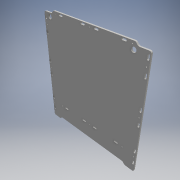
# Autodesk Inventor part: painel direito
Saved by Autodesk Inventor 2016 (Build 200138000, 138)
## iProperties
Created: 2016-08-08
Part Number: painel direito
Material: Generic
Document SubType Name: Modeling
Designer: Waldo
Density: 1 g/cm^3
Appearance: Default
Author: Waldo
Autodesk Inventor part; units mm, degrees
ref_plane "YZ Plane" through (0, 0, 0) normal (1, 0, 0) x (0, 1, 0)
ref_plane "XZ Plane" through (0, 0, 0) normal (0, 1, 0) x (-1, 0, 0)
ref_plane "XY Plane" through (0, 0, 0) normal (0, 0, 1) x (1, 0, 0)
sketch "Sketch1" plane through (0, 0, 0) normal (0, 1, 0) x (-1, 0, 0)
  line L0 (173.9968, 182.2069) -> (173.9968, 192.2069)
  arc A0 (167.7968, 182.2069) -> (173.9968, 182.2069) centre (170.8968, 182.2069) ccw
  line L1 (167.7968, 192.2069) -> (167.7968, 182.2069)
  arc A1 (173.9968, 192.2069) -> (167.7968, 192.2069) centre (170.8968, 192.2069) ccw
  line L2 (14.5968, -131.4908) -> (4.5968, -131.4908)
  arc A2 (14.5968, -137.6908) -> (14.5968, -131.4908) centre (14.5968, -134.5908) ccw
  line L3 (4.5968, -137.6908) -> (14.5968, -137.6908)
  arc A3 (4.5968, -131.4908) -> (4.5968, -137.6908) centre (4.5968, -134.5908) ccw
  line L4 (105.0968, -131.4908) -> (95.0968, -131.4908)
  arc A4 (105.0968, -137.6908) -> (105.0968, -131.4908) centre (105.0968, -134.5908) ccw
  line L5 (95.0968, -137.6908) -> (105.0968, -137.6908)
  arc A5 (95.0968, -131.4908) -> (95.0968, -137.6908) centre (95.0968, -134.5908) ccw
  line L6 (-135.9032, -137.6908) -> (-125.9032, -137.6908)
  arc A6 (-135.9032, -131.4908) -> (-135.9032, -137.6908) centre (-135.9032, -134.5908) ccw
  line L7 (-125.9032, -131.4908) -> (-135.9032, -131.4908)
  arc A7 (-125.9032, -137.6908) -> (-125.9032, -131.4908) centre (-125.9032, -134.5908) ccw
  line L8 (-45.4032, -137.6908) -> (-35.4032, -137.6908)
  arc A8 (-45.4032, -131.4908) -> (-45.4032, -137.6908) centre (-45.4032, -134.5908) ccw
  line L9 (-35.4032, -131.4908) -> (-45.4032, -131.4908)
  arc A9 (-35.4032, -137.6908) -> (-35.4032, -131.4908) centre (-35.4032, -134.5908) ccw
  line L10 (14.5968, 210.5092) -> (4.5968, 210.5092)
  arc A10 (14.5968, 204.3092) -> (14.5968, 210.5092) centre (14.5968, 207.4092) ccw
  line L11 (4.5968, 204.3092) -> (14.5968, 204.3092)
  arc A11 (4.5968, 210.5092) -> (4.5968, 204.3092) centre (4.5968, 207.4092) ccw
  line L12 (105.0968, 210.5092) -> (95.0968, 210.5092)
  arc A12 (105.0968, 204.3092) -> (105.0968, 210.5092) centre (105.0968, 207.4092) ccw
  line L13 (95.0968, 204.3092) -> (105.0968, 204.3092)
  arc A13 (95.0968, 210.5092) -> (95.0968, 204.3092) centre (95.0968, 207.4092) ccw
  line L14 (-135.9032, 204.3092) -> (-125.9032, 204.3092)
  arc A14 (-135.9032, 210.5092) -> (-135.9032, 204.3092) centre (-135.9032, 207.4092) ccw
  line L15 (-125.9032, 210.5092) -> (-135.9032, 210.5092)
  arc A15 (-125.9032, 204.3092) -> (-125.9032, 210.5092) centre (-125.9032, 207.4092) ccw
  line L16 (-45.4032, 204.3092) -> (-35.4032, 204.3092)
  arc A16 (-45.4032, 210.5092) -> (-45.4032, 204.3092) centre (-45.4032, 207.4092) ccw
  line L17 (-35.4032, 210.5092) -> (-45.4032, 210.5092)
  arc A17 (-35.4032, 204.3092) -> (-35.4032, 210.5092) centre (-35.4032, 207.4092) ccw
  line L18 (173.9968, 132.2069) -> (173.9968, 142.2069)
  arc A18 (167.7968, 132.2069) -> (173.9968, 132.2069) centre (170.8968, 132.2069) ccw
  line L19 (167.7968, 142.2069) -> (167.7968, 132.2069)
  arc A19 (173.9968, 142.2069) -> (167.7968, 142.2069) centre (170.8968, 142.2069) ccw
  line L20 (173.9968, 29.7671) -> (173.9968, 39.7671)
  arc A20 (167.7968, 29.7671) -> (173.9968, 29.7671) centre (170.8968, 29.7671) ccw
  line L21 (167.7968, 39.7671) -> (167.7968, 29.7671)
  arc A21 (173.9968, 39.7671) -> (167.7968, 39.7671) centre (170.8968, 39.7671) ccw
  line L22 (173.9968, -21.9484) -> (173.9968, -11.9484)
  arc A22 (167.7968, -21.9484) -> (173.9968, -21.9484) centre (170.8968, -21.9484) ccw
  line L23 (167.7968, -11.9484) -> (167.7968, -21.9484)
  arc A23 (173.9968, -11.9484) -> (167.7968, -11.9484) centre (170.8968, -11.9484) ccw
  line L24 (173.9968, -124.3882) -> (173.9968, -114.3882)
  arc A24 (167.7968, -124.3882) -> (173.9968, -124.3882) centre (170.8968, -124.3882) ccw
  line L25 (167.7968, -114.3882) -> (167.7968, -124.3882)
  arc A25 (173.9968, -114.3882) -> (167.7968, -114.3882) centre (170.8968, -114.3882) ccw
  line L26 (173.9968, -174.3882) -> (173.9968, -164.3882)
  arc A26 (167.7968, -174.3882) -> (173.9968, -174.3882) centre (170.8968, -174.3882) ccw
  line L27 (167.7968, -164.3882) -> (167.7968, -174.3882)
  arc A27 (173.9968, -164.3882) -> (167.7968, -164.3882) centre (170.8968, -164.3882) ccw
  line L28 (-204.8032, -11.9484) -> (-204.8032, -21.9484)
  arc A28 (-198.6032, -11.9484) -> (-204.8032, -11.9484) centre (-201.7032, -11.9484) ccw
  line L29 (-198.6032, -21.9484) -> (-198.6032, -11.9484)
  arc A29 (-204.8032, -21.9484) -> (-198.6032, -21.9484) centre (-201.7032, -21.9484) ccw
  line L30 (-204.8032, 39.7671) -> (-204.8032, 29.7671)
  arc A30 (-198.6032, 39.7671) -> (-204.8032, 39.7671) centre (-201.7032, 39.7671) ccw
  line L31 (-198.6032, 29.7671) -> (-198.6032, 39.7671)
  arc A31 (-204.8032, 29.7671) -> (-198.6032, 29.7671) centre (-201.7032, 29.7671) ccw
  line L32 (-204.8032, -164.3882) -> (-204.8032, -174.3882)
  arc A32 (-198.6032, -164.3882) -> (-204.8032, -164.3882) centre (-201.7032, -164.3882) ccw
  line L33 (-198.6032, -174.3882) -> (-198.6032, -164.3882)
  arc A33 (-204.8032, -174.3882) -> (-198.6032, -174.3882) centre (-201.7032, -174.3882) ccw
  line L34 (-204.8032, -114.3882) -> (-204.8032, -124.3882)
  arc A34 (-198.6032, -114.3882) -> (-204.8032, -114.3882) centre (-201.7032, -114.3882) ccw
  line L35 (-198.6032, -124.3882) -> (-198.6032, -114.3882)
  arc A35 (-204.8032, -124.3882) -> (-198.6032, -124.3882) centre (-201.7032, -124.3882) ccw
  line L36 (-204.8032, 142.2069) -> (-204.8032, 132.2069)
  arc A36 (-198.6032, 142.2069) -> (-204.8032, 142.2069) centre (-201.7032, 142.2069) ccw
  line L37 (-198.6032, 132.2069) -> (-198.6032, 142.2069)
  arc A37 (-204.8032, 132.2069) -> (-198.6032, 132.2069) centre (-201.7032, 132.2069) ccw
  line L38 (-204.8032, 192.2069) -> (-204.8032, 182.2069)
  arc A38 (-198.6032, 192.2069) -> (-204.8032, 192.2069) centre (-201.7032, 192.2069) ccw
  line L39 (-198.6032, 182.2069) -> (-198.6032, 192.2069)
  arc A39 (-204.8032, 182.2069) -> (-198.6032, 182.2069) centre (-201.7032, 182.2069) ccw
  circle A40 centre (151.4968, 191.5069) radius 8
  circle A41 centre (-160.6032, 191.5069) radius 8
  arc A42 (135.2533, -199.1268) -> (128.7419, -196.0905) centre (128.7419, -204.5905) ccw
  line L40 (135.2533, -199.1268) -> (138.549, -203.0545)
  arc A43 (138.549, -203.0545) -> (145.0604, -206.0908) centre (145.0604, -197.5908) ccw
  line L41 (145.0604, -206.0908) -> (171.0968, -206.0908)
  arc A44 (171.0968, -206.0908) -> (177.0968, -200.0908) centre (171.0968, -200.0908) ccw
  line L42 (177.0968, -200.0908) -> (177.0968, 198.0069)
  arc A45 (177.0968, 198.0069) -> (171.0968, 204.0069) centre (171.0968, 198.0069) ccw
  line L43 (171.0968, 204.0069) -> (145.0968, 204.0069)
  arc A46 (138.5854, 207.0432) -> (145.0968, 204.0069) centre (145.0968, 212.5069) ccw
  line L44 (138.5854, 207.0432) -> (135.3719, 210.8729)
  arc A47 (135.3719, 210.8729) -> (128.8605, 213.9092) centre (128.8605, 205.4092) ccw
  line L45 (128.8605, 213.9092) -> (-159.667, 213.9092)
  arc A48 (-159.667, 213.9092) -> (-166.1784, 210.8729) centre (-159.667, 205.4092) ccw
  line L46 (-166.1784, 210.8729) -> (-169.3918, 207.0432)
  arc A49 (-175.9032, 204.0069) -> (-169.3918, 207.0432) centre (-175.9032, 212.5069) ccw
  line L47 (-175.9032, 204.0069) -> (-201.9032, 204.0069)
  arc A50 (-201.9032, 204.0069) -> (-207.9032, 198.0069) centre (-201.9032, 198.0069) ccw
  line L48 (-207.9032, 198.0069) -> (-207.9032, -200.0908)
  arc A51 (-207.9032, -200.0908) -> (-201.9032, -206.0908) centre (-201.9032, -200.0908) ccw
  line L49 (-201.9032, -206.0908) -> (-175.8668, -206.0908)
  arc A52 (-175.8668, -206.0908) -> (-169.3555, -203.0545) centre (-175.8668, -197.5908) ccw
  line L50 (-169.3555, -203.0545) -> (-166.0597, -199.1268)
  arc A53 (-159.5483, -196.0905) -> (-166.0597, -199.1268) centre (-159.5483, -204.5905) ccw
  line L51 (-159.5483, -196.0905) -> (128.7419, -196.0905)
  circle A54 centre (-15.4032, 205.9092) radius 1.55
  circle A55 centre (125.0968, 205.9092) radius 1.55
  circle A56 centre (-155.9032, 205.9092) radius 1.55
  circle A57 centre (-15.4032, -136.0908) radius 1.55
  circle A58 centre (125.0968, -136.0908) radius 1.55
  circle A59 centre (-155.9032, -136.0908) radius 1.55
  circle A60 centre (-200.1532, 162.2069) radius 1.6
  circle A61 centre (-200.1532, 8.9094) radius 1.6
  circle A62 centre (-200.1532, -144.3882) radius 1.6
  circle A63 centre (169.3468, -144.3882) radius 1.6
  circle A64 centre (169.3468, 8.9094) radius 1.6
  circle A65 centre (169.3468, 162.2069) radius 1.6
  point P0 (0, 0)
  constraints: 130 tangent, 104 end point, 104 point on circle, 66 centre point, 60 equal radius, 12 parallel, 8 perpendicular, 1 collinear
extrude "Extrusion1" add sketch "Sketch1" along normal blind 6
body "Solid1"
